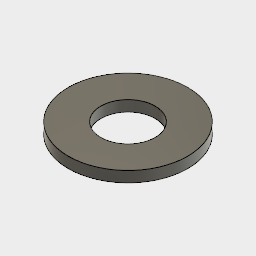
Washer M10 20mm 2mm (Autodesk Fusion 360 design; units mm, degrees)
Autodesk Fusion 360 part; units mm, degrees
sketch "Skizze1" plane through (0, 0, 0) normal (0, 1, 0) x (1, 0, 0)
  circle A0 centre (0, 0) radius 5
  circle A1 centre (0, 0) radius 11
  dimension "d1" = 10
  dimension "d2" = 22
  measures "d1" diameter of A0
  measures "d2" diameter of A1
extrude "Extrusion2" add sketch "Skizze1" along normal blind 2
